Autodesk Inventor part; units mm, degrees
(part 2 of 2)
sketch "Sketch17" plane through (0, 3.175, 0) normal (0, 1, 0) x (1, 0, 0)
  line L0 (-195.7502, -16.6805) -> (-149.2548, -16.6805) construction
  line L1 (-149.2548, -16.6805) -> (-149.2548, -30.1673) construction
  line L2 (-149.2548, -30.1673) -> (-195.7502, -30.1673) construction
  line L3 (-195.7502, -30.1673) -> (-195.7502, -16.6805) construction
  line L4 (-200.8302, -13.1267) -> (-200.8302, -33.721) projected
  line L5 (-200.8302, -23.4239) -> (-144.5457, -23.4239) construction
  line L6 (-192.2947, -27.1971) -> (-192.2947, -19.7535)
  line L7 (-192.2947, -19.7535) -> (-190.972, -19.658)
  spline S0 degree 2 poles (-190.972, -19.658) (-190.0682, -19.658) (-189.5097, -20.2458) knots 0 0 0 1 1 1
  spline S1 degree 2 poles (-189.5097, -20.2458) (-188.966, -20.8337) (-188.966, -21.7228) knots 0 0 0 1 1 1
  spline S2 degree 2 poles (-188.966, -21.7228) (-188.966, -22.847) (-189.8845, -23.1777) knots 0 0 0 1 1 1
  spline S3 degree 2 poles (-189.8845, -23.1777) (-188.4075, -23.4496) (-188.4075, -25.1397) knots 0 0 0 1 1 1
  spline S4 degree 2 poles (-188.4075, -25.1397) (-188.4075, -25.9847) (-188.9292, -26.624) knots 0 0 0 1 1 1
  spline S5 degree 2 poles (-188.9292, -26.624) (-189.4583, -27.278) (-190.6193, -27.278) knots 0 0 0 1 1 1
  spline S6 degree 2 poles (-190.6193, -27.278) (-191.0308, -27.278) (-191.5011, -27.2339) knots 0 0 0 1 1 1
  spline S7 degree 2 poles (-191.5011, -27.2339) (-191.9273, -27.1971) (-192.2947, -27.1971) knots 0 0 0 1 1 1
  line L8 (-192.5151, -19.7461) -> (-192.5151, -27.1898)
  spline S8 degree 2 poles (-192.5151, -27.1898) (-193.2426, -27.2192) (-194.2346, -27.278) knots 0 0 0 1 1 1
  line L9 (-194.2346, -27.278) -> (-194.2346, -26.9105)
  spline S9 degree 2 poles (-194.2346, -26.9105) (-193.3601, -26.6681) (-193.3601, -25.169) knots 0 0 0 1 1 1
  line L10 (-193.3601, -25.169) -> (-193.3601, -21.6199)
  spline S10 degree 2 poles (-193.3601, -21.6199) (-193.3601, -20.3119) (-194.2346, -20.0254) knots 0 0 0 1 1 1
  line L11 (-194.2346, -20.0254) -> (-194.2346, -19.658)
  spline S11 degree 2 poles (-194.2346, -19.658) (-193.3675, -19.7241) (-192.5151, -19.7461) knots 0 0 0 1 1 1
  line L12 (-190.9132, -23.7288) -> (-191.4496, -23.7288)
  line L13 (-191.4496, -23.7288) -> (-191.4496, -24.8163)
  spline S12 degree 2 poles (-191.4496, -24.8163) (-191.4496, -26.0582) (-191.2145, -26.3447) knots 0 0 0 1 1 1
  spline S13 degree 2 poles (-191.2145, -26.3447) (-191.0308, -26.4844) (-190.6046, -26.4844) knots 0 0 0 1 1 1
  spline S14 degree 2 poles (-190.6046, -26.4844) (-189.8771, -26.4844) (-189.5979, -26.1023) knots 0 0 0 1 1 1
  spline S15 degree 2 poles (-189.5979, -26.1023) (-189.2819, -25.654) (-189.2819, -25.0809) knots 0 0 0 1 1 1
  spline S16 degree 2 poles (-189.2819, -25.0809) (-189.2819, -24.6253) (-189.3701, -24.3681) knots 0 0 0 1 1 1
  spline S17 degree 2 poles (-189.3701, -24.3681) (-189.6714, -23.9786) (-189.9433, -23.8611) knots 0 0 0 1 1 1
  spline S18 degree 2 poles (-189.9433, -23.8611) (-190.2739, -23.7288) (-190.9132, -23.7288) knots 0 0 0 1 1 1
  line L14 (-191.4496, -21.7375) -> (-191.4496, -22.9646)
  line L15 (-191.4496, -22.9646) -> (-191.0749, -22.9646)
  spline S19 degree 2 poles (-191.0749, -22.9646) (-190.4797, -22.9646) (-190.1711, -22.656) knots 0 0 0 1 1 1
  spline S20 degree 2 poles (-190.1711, -22.656) (-189.8551, -22.34) (-189.8551, -21.7301) knots 0 0 0 1 1 1
  spline S21 degree 2 poles (-189.8551, -21.7301) (-189.8551, -21.1129) (-190.2372, -20.694) knots 0 0 0 1 1 1
  spline S22 degree 2 poles (-190.2372, -20.694) (-190.5311, -20.4736) (-191.0014, -20.4736) knots 0 0 0 1 1 1
  spline S23 degree 2 poles (-191.0014, -20.4736) (-191.2439, -20.4736) (-191.3468, -20.5618) knots 0 0 0 1 1 1
  spline S24 degree 2 poles (-191.3468, -20.5618) (-191.4496, -20.863) (-191.4496, -21.7375) knots 0 0 0 1 1 1
  spline S25 degree 2 poles (-188.819, -27.0061) (-188.1871, -26.1463) (-188.1871, -25.1764) knots 0 0 0 1 1 1
  spline S26 degree 2 poles (-188.1871, -25.1764) (-188.1871, -24.133) (-188.8484, -23.2512) knots 0 0 0 1 1 1
  spline S27 degree 2 poles (-188.8484, -23.2512) (-187.2612, -23.7656) (-187.2612, -25.1176) knots 0 0 0 1 1 1
  spline S28 degree 2 poles (-187.2612, -25.1176) (-187.2612, -25.7863) (-187.6507, -26.308) knots 0 0 0 1 1 1
  spline S29 degree 2 poles (-187.6507, -26.308) (-188.0401, -26.8297) (-188.819, -27.0061) knots 0 0 0 1 1 1
  spline S30 degree 2 poles (-189.157, -23.1483) (-188.7455, -22.4208) (-188.7455, -21.7154) knots 0 0 0 1 1 1
  spline S31 degree 2 poles (-188.7455, -21.7154) (-188.7455, -21.1643) (-188.9586, -20.7234) knots 0 0 0 1 1 1
  spline S32 degree 2 poles (-188.9586, -20.7234) (-189.1791, -20.2752) (-189.5244, -19.871) knots 0 0 0 1 1 1
  spline S33 degree 2 poles (-189.5244, -19.871) (-188.628, -20.0327) (-188.2385, -20.503) knots 0 0 0 1 1 1
  spline S34 degree 2 poles (-188.2385, -20.503) (-187.8417, -20.988) (-187.8417, -21.5685) knots 0 0 0 1 1 1
  spline S35 degree 2 poles (-187.8417, -21.5685) (-187.8417, -22.0902) (-188.1503, -22.5237) knots 0 0 0 1 1 1
  spline S36 degree 2 poles (-188.1503, -22.5237) (-188.4957, -22.994) (-189.157, -23.1483) knots 0 0 0 1 1 1
  spline S37 degree 2 poles (-179.2003, -23.4275) (-179.2003, -24.7135) (-179.5971, -25.6099) knots 0 0 0 1 1 1
  spline S38 degree 2 poles (-179.5971, -25.6099) (-179.9866, -26.5064) (-180.6479, -26.8959) knots 0 0 0 1 1 1
  spline S39 degree 2 poles (-180.6479, -26.8959) (-181.4048, -27.3735) (-182.3453, -27.3735) knots 0 0 0 1 1 1
  spline S40 degree 2 poles (-182.3453, -27.3735) (-183.8296, -27.3735) (-184.6526, -26.3007) knots 0 0 0 1 1 1
  spline S41 degree 2 poles (-184.6526, -26.3007) (-185.4536, -25.2499) (-185.4536, -23.4202) knots 0 0 0 1 1 1
  spline S42 degree 2 poles (-185.4536, -23.4202) (-185.4536, -21.5244) (-184.6379, -20.503) knots 0 0 0 1 1 1
  spline S43 degree 2 poles (-184.6379, -20.503) (-183.8002, -19.4742) (-182.36, -19.4742) knots 0 0 0 1 1 1
  spline S44 degree 2 poles (-182.36, -19.4742) (-180.8904, -19.4742) (-180.038, -20.503) knots 0 0 0 1 1 1
  spline S45 degree 2 poles (-180.038, -20.503) (-179.2003, -21.5097) (-179.2003, -23.4275) knots 0 0 0 1 1 1
  spline S46 degree 2 poles (-180.1262, -23.4349) (-180.1262, -20.3119) (-182.36, -20.3119) knots 0 0 0 1 1 1
  spline S47 degree 2 poles (-182.36, -20.3119) (-184.5351, -20.3119) (-184.5351, -23.5157) knots 0 0 0 1 1 1
  spline S48 degree 2 poles (-184.5351, -23.5157) (-184.5351, -26.5284) (-182.3306, -26.5284) knots 0 0 0 1 1 1
  spline S49 degree 2 poles (-182.3306, -26.5284) (-180.1262, -26.5284) (-180.1262, -23.4349) knots 0 0 0 1 1 1
  spline S50 degree 2 poles (-184.9392, -20.3707) (-185.6887, -21.7081) (-185.6887, -23.479) knots 0 0 0 1 1 1
  spline S51 degree 2 poles (-185.6887, -23.479) (-185.6887, -25.0809) (-184.9686, -26.455) knots 0 0 0 1 1 1
  spline S52 degree 2 poles (-184.9686, -26.455) (-186.6366, -25.485) (-186.6366, -23.4128) knots 0 0 0 1 1 1
  spline S53 degree 2 poles (-186.6366, -23.4128) (-186.6366, -21.2819) (-184.9392, -20.3707) knots 0 0 0 1 1 1
  spline S54 degree 2 poles (-179.7294, -26.4917) (-178.9946, -25.3013) (-178.9946, -23.3173) knots 0 0 0 1 1 1
  spline S55 degree 2 poles (-178.9946, -23.3173) (-178.9946, -21.5685) (-179.722, -20.3781) knots 0 0 0 1 1 1
  spline S56 degree 2 poles (-179.722, -20.3781) (-178.0393, -21.2819) (-178.0393, -23.3908) knots 0 0 0 1 1 1
  spline S57 degree 2 poles (-178.0393, -23.3908) (-178.0393, -25.463) (-179.7294, -26.4917) knots 0 0 0 1 1 1
  line L16 (-172.903, -27.1971) -> (-173.2189, -27.1971)
  line L17 (-173.2189, -27.1971) -> (-173.2189, -19.7388)
  line L18 (-173.2189, -19.7388) -> (-170.6251, -19.7388)
  spline S58 degree 2 poles (-170.6251, -19.7388) (-169.949, -19.7388) (-169.1481, -19.658) knots 0 0 0 1 1 1
  spline S59 degree 2 poles (-169.1481, -19.658) (-169.1481, -19.8931) (-169.1701, -20.2752) knots 0 0 0 1 1 1
  spline S60 degree 2 poles (-169.1701, -20.2752) (-169.1922, -20.5544) (-169.1922, -21.0541) knots 0 0 0 1 1 1
  spline S61 degree 2 poles (-169.1922, -21.0541) (-169.1922, -21.348) (-169.2436, -21.7963) knots 0 0 0 1 1 1
  line L19 (-169.2436, -21.7963) -> (-169.6698, -21.7963)
  spline S62 degree 2 poles (-169.6698, -21.7963) (-169.6845, -21.1496) (-169.927, -20.8116) knots 0 0 0 1 1 1
  spline S63 degree 2 poles (-169.927, -20.8116) (-170.1621, -20.4956) (-170.9704, -20.4956) knots 0 0 0 1 1 1
  line L20 (-170.9704, -20.4956) -> (-172.3666, -20.4956)
  line L21 (-172.3666, -20.4956) -> (-172.3666, -25.2278)
  spline S64 degree 2 poles (-172.3666, -25.2278) (-172.3666, -26.0361) (-172.1461, -26.4182) knots 0 0 0 1 1 1
  spline S65 degree 2 poles (-172.1461, -26.4182) (-171.9404, -26.793) (-171.3893, -26.9032) knots 0 0 0 1 1 1
  line L22 (-171.3893, -26.9032) -> (-171.3893, -27.278)
  spline S66 degree 2 poles (-171.3893, -27.278) (-172.756, -27.1971) (-172.903, -27.1971) knots 0 0 0 1 1 1
  line L23 (-175.8937, -19.7388) -> (-173.4394, -19.7388)
  line L24 (-173.4394, -19.7388) -> (-173.4394, -27.1971)
  line L25 (-173.4394, -27.1971) -> (-173.7921, -27.1971)
  spline S67 degree 2 poles (-173.7921, -27.1971) (-174.2183, -27.1971) (-175.2544, -27.278) knots 0 0 0 1 1 1
  line L26 (-175.2544, -27.278) -> (-175.2544, -26.9032)
  spline S68 degree 2 poles (-175.2544, -26.9032) (-174.6445, -26.7489) (-174.4608, -26.3741) knots 0 0 0 1 1 1
  spline S69 degree 2 poles (-174.4608, -26.3741) (-174.2697, -25.9773) (-174.2697, -25.0074) knots 0 0 0 1 1 1
  line L27 (-174.2697, -25.0074) -> (-174.2697, -20.4956)
  line L28 (-174.2697, -20.4956) -> (-175.8643, -20.4956)
  spline S70 degree 2 poles (-175.8643, -20.4956) (-176.4668, -20.4956) (-176.6946, -20.7308) knots 0 0 0 1 1 1
  spline S71 degree 2 poles (-176.6946, -20.7308) (-176.9371, -20.9733) (-177.1428, -21.7963) knots 0 0 0 1 1 1
  line L29 (-177.1428, -21.7963) -> (-177.547, -21.7963)
  spline S72 degree 2 poles (-177.547, -21.7963) (-177.5617, -21.5758) (-177.5617, -21.4656) knots 0 0 0 1 1 1
  spline S73 degree 2 poles (-177.5617, -21.4656) (-177.5617, -21.3113) (-177.5323, -21.0908) knots 0 0 0 1 1 1
  spline S74 degree 2 poles (-177.5323, -21.0908) (-177.4515, -20.3707) (-177.4515, -19.658) knots 0 0 0 1 1 1
  spline S75 degree 2 poles (-177.4515, -19.658) (-176.9297, -19.7094) (-176.3933, -19.7241) knots 0 0 0 1 1 1
  line L30 (-176.3933, -19.7241) -> (-175.8937, -19.7388)
  line L31 (-164.144, -27.1971) -> (-164.46, -27.1971)
  line L32 (-164.46, -27.1971) -> (-164.46, -19.7388)
  line L33 (-164.46, -19.7388) -> (-161.8661, -19.7388)
  spline S76 degree 2 poles (-161.8661, -19.7388) (-161.1901, -19.7388) (-160.3891, -19.658) knots 0 0 0 1 1 1
  spline S77 degree 2 poles (-160.3891, -19.658) (-160.3891, -19.8931) (-160.4112, -20.2752) knots 0 0 0 1 1 1
  spline S78 degree 2 poles (-160.4112, -20.2752) (-160.4332, -20.5544) (-160.4332, -21.0541) knots 0 0 0 1 1 1
  spline S79 degree 2 poles (-160.4332, -21.0541) (-160.4332, -21.348) (-160.4847, -21.7963) knots 0 0 0 1 1 1
  line L34 (-160.4847, -21.7963) -> (-160.9108, -21.7963)
  spline S80 degree 2 poles (-160.9108, -21.7963) (-160.9255, -21.1496) (-161.168, -20.8116) knots 0 0 0 1 1 1
  spline S81 degree 2 poles (-161.168, -20.8116) (-161.4032, -20.4956) (-162.2115, -20.4956) knots 0 0 0 1 1 1
  line L35 (-162.2115, -20.4956) -> (-163.6076, -20.4956)
  line L36 (-163.6076, -20.4956) -> (-163.6076, -25.2278)
  spline S82 degree 2 poles (-163.6076, -25.2278) (-163.6076, -26.0361) (-163.3872, -26.4182) knots 0 0 0 1 1 1
  spline S83 degree 2 poles (-163.3872, -26.4182) (-163.1814, -26.793) (-162.6303, -26.9032) knots 0 0 0 1 1 1
  line L37 (-162.6303, -26.9032) -> (-162.6303, -27.278)
  spline S84 degree 2 poles (-162.6303, -27.278) (-163.9971, -27.1971) (-164.144, -27.1971) knots 0 0 0 1 1 1
  line L38 (-167.1347, -19.7388) -> (-164.6804, -19.7388)
  line L39 (-164.6804, -19.7388) -> (-164.6804, -27.1971)
  line L40 (-164.6804, -27.1971) -> (-165.0331, -27.1971)
  spline S85 degree 2 poles (-165.0331, -27.1971) (-165.4593, -27.1971) (-166.4954, -27.278) knots 0 0 0 1 1 1
  line L41 (-166.4954, -27.278) -> (-166.4954, -26.9032)
  spline S86 degree 2 poles (-166.4954, -26.9032) (-165.8855, -26.7489) (-165.7018, -26.3741) knots 0 0 0 1 1 1
  spline S87 degree 2 poles (-165.7018, -26.3741) (-165.5108, -25.9773) (-165.5108, -25.0074) knots 0 0 0 1 1 1
  line L42 (-165.5108, -25.0074) -> (-165.5108, -20.4956)
  line L43 (-165.5108, -20.4956) -> (-167.1053, -20.4956)
  spline S88 degree 2 poles (-167.1053, -20.4956) (-167.7079, -20.4956) (-167.9357, -20.7308) knots 0 0 0 1 1 1
  spline S89 degree 2 poles (-167.9357, -20.7308) (-168.1781, -20.9733) (-168.3839, -21.7963) knots 0 0 0 1 1 1
  line L44 (-168.3839, -21.7963) -> (-168.788, -21.7963)
  spline S90 degree 2 poles (-168.788, -21.7963) (-168.8027, -21.5758) (-168.8027, -21.4656) knots 0 0 0 1 1 1
  spline S91 degree 2 poles (-168.8027, -21.4656) (-168.8027, -21.3113) (-168.7733, -21.0908) knots 0 0 0 1 1 1
  spline S92 degree 2 poles (-168.7733, -21.0908) (-168.6925, -20.3707) (-168.6925, -19.658) knots 0 0 0 1 1 1
  spline S93 degree 2 poles (-168.6925, -19.658) (-168.1708, -19.7094) (-167.6344, -19.7241) knots 0 0 0 1 1 1
  line L45 (-167.6344, -19.7241) -> (-167.1347, -19.7388)
  line L46 (-154.7237, -27.1971) -> (-154.7237, -23.4863)
  line L47 (-154.7237, -23.4863) -> (-158.1333, -19.7388)
  line L48 (-158.1333, -19.7388) -> (-157.8026, -19.7388)
  spline S94 degree 2 poles (-157.8026, -19.7388) (-156.987, -19.7388) (-155.9803, -19.658) knots 0 0 0 1 1 1
  line L49 (-155.9803, -19.658) -> (-155.9803, -20.0254)
  spline S95 degree 2 poles (-155.9803, -20.0254) (-156.3844, -20.1429) (-156.3844, -20.3046) knots 0 0 0 1 1 1
  spline S96 degree 2 poles (-156.3844, -20.3046) (-156.3844, -20.6059) (-155.6055, -21.4142) knots 0 0 0 1 1 1
  line L50 (-155.6055, -21.4142) -> (-154.2755, -22.8691)
  line L51 (-154.2755, -22.8691) -> (-153.0337, -21.348)
  spline S97 degree 2 poles (-153.0337, -21.348) (-152.6148, -20.863) (-152.6148, -20.503) knots 0 0 0 1 1 1
  spline S98 degree 2 poles (-152.6148, -20.503) (-152.6148, -20.1429) (-153.0851, -20.0327) knots 0 0 0 1 1 1
  line L52 (-153.0851, -20.0327) -> (-153.0851, -19.658)
  spline S99 degree 2 poles (-153.0851, -19.658) (-152.7985, -19.658) (-152.0858, -19.7094) knots 0 0 0 1 1 1
  spline S100 degree 2 poles (-152.0858, -19.7094) (-151.8433, -19.7388) (-151.6228, -19.7388) knots 0 0 0 1 1 1
  spline S101 degree 2 poles (-151.6228, -19.7388) (-151.4906, -19.7388) (-150.2781, -19.658) knots 0 0 0 1 1 1
  line L53 (-150.2781, -19.658) -> (-150.2781, -20.0254)
  spline S102 degree 2 poles (-150.2781, -20.0254) (-150.866, -20.1944) (-151.1672, -20.4515) knots 0 0 0 1 1 1
  spline S103 degree 2 poles (-151.1672, -20.4515) (-151.4538, -20.7014) (-151.8286, -21.1496) knots 0 0 0 1 1 1
  spline S104 degree 2 poles (-151.8286, -21.1496) (-151.858, -21.2011) (-151.9682, -21.3186) knots 0 0 0 1 1 1
  line L54 (-151.9682, -21.3186) -> (-153.886, -23.5672)
  line L55 (-153.886, -23.5672) -> (-153.886, -25.2425)
  spline S105 degree 2 poles (-153.886, -25.2425) (-153.886, -26.7048) (-152.9087, -26.9032) knots 0 0 0 1 1 1
  line L56 (-152.9087, -26.9032) -> (-152.9087, -27.278)
  spline S106 degree 2 poles (-152.9087, -27.278) (-154.3122, -27.1971) (-154.3416, -27.1971) knots 0 0 0 1 1 1
  line L57 (-154.3416, -27.1971) -> (-154.7237, -27.1971)
  line L58 (-158.5888, -19.7388) -> (-154.9662, -23.5745)
  line L59 (-154.9662, -23.5745) -> (-154.9662, -27.1971)
  line L60 (-154.9662, -27.1971) -> (-155.2748, -27.1971)
  spline S107 degree 2 poles (-155.2748, -27.1971) (-155.8553, -27.1971) (-156.7886, -27.278) knots 0 0 0 1 1 1
  line L61 (-156.7886, -27.278) -> (-156.7886, -26.9032)
  spline S108 degree 2 poles (-156.7886, -26.9032) (-156.2815, -26.7856) (-156.0537, -26.4844) knots 0 0 0 1 1 1
  spline S109 degree 2 poles (-156.0537, -26.4844) (-155.8259, -26.1831) (-155.8259, -25.2719) knots 0 0 0 1 1 1
  line L62 (-155.8259, -25.2719) -> (-155.8259, -23.839)
  line L63 (-155.8259, -23.839) -> (-157.9569, -21.5905)
  spline S110 degree 2 poles (-157.9569, -21.5905) (-159.1693, -20.3193) (-160.2348, -20.0327) knots 0 0 0 1 1 1
  line L64 (-160.2348, -20.0327) -> (-160.2348, -19.658)
  spline S111 degree 2 poles (-160.2348, -19.658) (-159.5221, -19.7388) (-158.8681, -19.7388) knots 0 0 0 1 1 1
  line L65 (-158.8681, -19.7388) -> (-158.5888, -19.7388)
  point P0 (0, 0)
  point P1 (-195.7502, -23.4239)
  dimension "d206" = 5.08
  constraints: 2 end point, 2 midpoint, 1 horizontal, 1 point on line, 2 other
  measures "d206" distance between parallel lines of L4 L3
emboss "Emboss2" sketch "Sketch17" operation add depth 0.4 direction (0, -1, 0)
sketch "Sketch13" plane through (0, 3.175, 0) normal (0, 1, 0) x (1, 0, 0)
  line L0 (-100.2262, -38.2104) -> (-100.2262, -157.352) construction
  line L1 (-100.2262, -157.352) -> (-143.0309, -157.352) construction
  line L2 (-143.0309, -157.352) -> (-143.0309, -38.2104) construction
  line L3 (-143.0309, -38.2104) -> (-100.2262, -38.2104) construction
  line L4 (-144.2491, -33.721) -> (-144.2491, -142.941) projected
  point P0 (0, 0)
  constraints: 1 parallel, 2 other
equation "\"d11\" = d9"
equation "\"d12\" = d10"
equation "\"d53\" = d11"
equation "\"d9\" = 144.1069"
body "Solid1"
